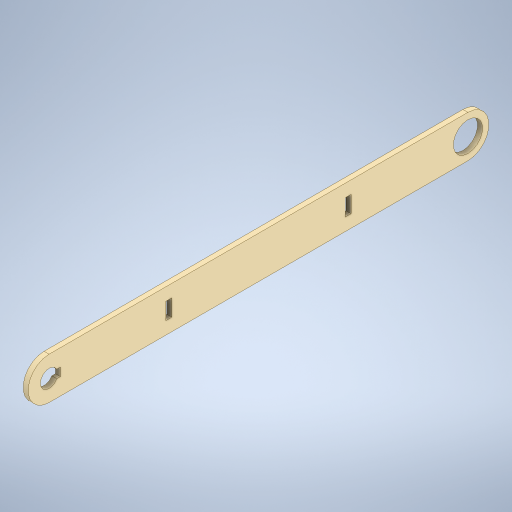
# Autodesk Inventor part: brazo3
Saved by Autodesk Inventor 2024.3 (Build 283343000, 343)
## iProperties
Created: 2024-05-14
Part Number: brazo3
Material: PMMA Plastic
Document SubType Name: Modeling
Designer: USUARIO
Density: 1.188 g/cm^3
Appearance: Beige
Mass: 22.2023 g
Surface Area: 144.043 cm^2
Volume: 18.6888 cm^3
Author: USUARIO
Autodesk Inventor part; units mm, degrees
ref_plane "YZ Plane" through (0, 0, 0) normal (1, 0, 0) x (0, 1, 0)
ref_plane "XZ Plane" through (0, 0, 0) normal (0, 1, 0) x (-1, 0, 0)
ref_plane "XY Plane" through (0, 0, 0) normal (0, 0, 1) x (1, 0, 0)
sketch "Sketch1" plane through (0, 0, 0) normal (1, 0, 0) x (0, 1, 0)
  line L0 (0, 0) -> (0, -250) construction
  circle A0 centre (0, -250) radius 8.75
  arc A1 (0, -12.5) -> (12.5, 0) centre (0, 0) ccw construction
  arc A2 (0, -237.5) -> (-12.5, -250) centre (0, -250) ccw construction
  line L1 (12.5, 0) -> (12.5, -250)
  line L2 (-12.5, 0) -> (-12.5, -250)
  arc A3 (-12.5, 0) -> (0, -12.5) centre (0, 0) ccw construction
  arc A4 (12.5, 0) -> (-12.5, 0) centre (0, 0) ccw
  arc A5 (12.5, -250) -> (0, -237.5) centre (0, -250) ccw construction
  arc A6 (-12.5, -250) -> (12.5, -250) centre (0, -250) ccw
  line L3 (0, 0) -> (0, -70) construction
  line L4 (0, -70) -> (5, -70) construction
  line L5 (5, -70) -> (5, -73)
  line L6 (5, -73) -> (-5, -73) construction
  line L7 (-5, -73) -> (-5, -70)
  line L8 (-5, -70) -> (0, -70) construction
  line L9 (0, -250) -> (0, -180) construction
  line L10 (0, -180) -> (5, -180) construction
  line L11 (5, -180) -> (5, -177)
  line L12 (5, -177) -> (-5, -177) construction
  line L13 (-5, -177) -> (-5, -180)
  line L14 (0, -180) -> (-5, -180) construction
  line L15 (7.5, 0) -> (13.5, 0) construction
  arc A7 (2.5, -4.6165) -> (-2.5, -4.6165) centre (0, 0) ccw
  line L16 (0, -5.25) -> (2.5, -5.25) construction
  line L17 (2.5, -5.25) -> (-2.5, -5.25) construction
  line L18 (-2.5, -5.25) -> (-2.5, -6.75)
  line L19 (-2.5, -6.75) -> (2.5, -6.75)
  line L20 (2.5, -6.75) -> (2.5, -5.25)
  line L21 (2.5, -5.25) -> (2.5, -4.6165)
  line L22 (-2.5, -5.25) -> (-2.5, -4.6165)
  arc A8 (0, -5.25) -> (2.5, -4.6165) centre (0, 0) ccw construction
  arc A9 (-2.5, -4.6165) -> (0, -5.25) centre (0, 0) ccw construction
  line L23 (5, -73) -> (5, -73.25)
  line L24 (5, -73.25) -> (-5, -73.25)
  line L25 (-5, -73.25) -> (-5, -73)
  line L26 (-5, -70) -> (-5, -69.75)
  line L27 (-5, -69.75) -> (5, -69.75)
  line L28 (5, -69.75) -> (5, -70)
  line L29 (5, -177) -> (5, -176.75)
  line L30 (5, -176.75) -> (-5, -176.75)
  line L31 (-5, -176.75) -> (-5, -177)
  line L32 (-5, -180) -> (-5, -180.25)
  line L33 (-5, -180.25) -> (5, -180.25)
  line L34 (5, -180.25) -> (5, -180)
  dimension "d1" = 250
  dimension "d2" = 17.5
  dimension "d3" = 25
  dimension "d4" = 25
  dimension "d5" = 70
  dimension "d6" = 5
  dimension "d7" = 3
  dimension "d9" = 70
  dimension "d10" = 3
  dimension "d14" = 10
  dimension "d17" = 10.5
  dimension "d18" = 2.5
  dimension "d19" = 5
  dimension "d20" = 1.5
  dimension "d21" = 0.25
  dimension "d22" = 10
  dimension "d23" = 0.25
  dimension "d24" = 0.25
  dimension "d25" = 10
  dimension "d26" = 0.25
  dimension "d27" = 10
  dimension "d28" = 0.25
  dimension "d29" = 10
  dimension "d30" = 0.25
  dimension "d31" = 0.25
  dimension "d32" = 10
  dimension "d33" = 0.25
  constraints: 70 end point, 18 point on circle, 13 perpendicular, 12 point on line, 10 centre point, 6 tangent, 5 coincident, 5 vertical, 3 parallel, 2 horizontal, 1 midpoint
  measures "d1" distance of L0.start L0.end
  measures "d2" diameter of A0
  measures "d3" diameter of A1
  measures "d4" diameter of A2
  measures "d5" distance of L3.start L3.end
  measures "d6" distance of L3.end L4.end
  measures "d7" distance of L4.end L5.end
  measures "d9" distance of L9.start L9.end
  measures "d10" distance of L10.end L11.end
  measures "d14" distance of L5.end L6.end
  measures "d17" diameter of A7
  measures "d18" distance of L16.start L16.end
  measures "d19" distance of L19.end L18.end
  measures "d20" distance of L18.end L17.end
  measures "d21" distance of L5.end L23.end
  measures "d22" distance of L23.end L24.end
  measures "d23" distance of L24.end L6.end
  measures "d24" distance of L7.end L26.end
  measures "d25" distance of L26.end L27.end
  measures "d26" distance of L27.end L4.end
  measures "d27" distance of L11.end L12.end
  measures "d28" distance of L11.end L29.end
  measures "d29" distance of L29.end L30.end
  measures "d30" distance of L30.end L12.end
  measures "d31" distance of L13.end L32.end
  measures "d32" distance of L32.end L33.end
  measures "d33" distance of L33.end L10.end
extrude "Extrusion1" add sketch "Sketch1" along normal blind 3
body "Solid1"
